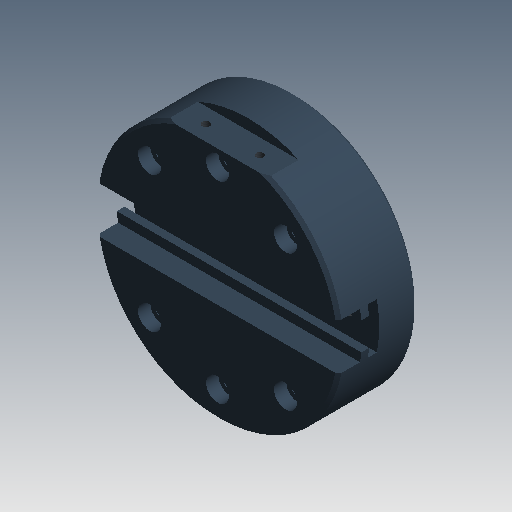
# Autodesk Inventor part: 210-101b
Saved by Autodesk Inventor 2020.1 (Build 241239000, 239)
## iProperties
Created: 2006-01-27
Part Number: 210-101b
Document SubType Name: Modeling
Designer: Kevin
Manufacturer: Standard
Standards Organization: Custom
Description: ADJUSTABLE CLAMP HEAD
Density: 1 g/cm^3
Material: Generic
Appearance: Grey - Blue Dark
Slot: 30.000 mm
Title: BLOCK
Author: Kevin
Revision Number: -
Autodesk Inventor part; units mm, degrees
ref_plane "YZ Plane" through (0, 0, 0) normal (1, 0, 0) x (0, 1, 0)
ref_plane "XZ Plane" through (0, 0, 0) normal (0, 1, 0) x (-1, 0, 0)
ref_plane "XY Plane" through (0, 0, 0) normal (0, 0, 1) x (1, 0, 0)
sketch "Sketch2" plane through (0, 0, 0) normal (0, 0, 1) x (1, 0, 0)
  circle A0 centre (0, 0) radius 80
  dimension "d0" = 160
  constraints: 1 centre point
  measures "d0" diameter of A0
extrude "Extrusion1" add sketch "Sketch2" along normal blind 50
sketch "Sketch7" plane through (0, 0, 50) normal (0, 0, 1) x (1, 0, 0)
  circle A0 centre (0, 0) radius 80 projected
  circle A1 centre (0, 0) radius 62.5 construction
  point P0 (0, 62.5)
  dimension "d48" = 125
  constraints: 2 vertical alignment, 1 coincident, 2 other
hole "Hole4" at (0, 62.5, 50) direction (0, 0, -1) diameter 9 end through all counterbore diameter 15 counterbore depth 8 clearance for "Socket Head Cap Screw" size "M8" standard "Ansi Metric M Profile"
pattern_circular "Circular Pattern2" count 8 over 360 about axis through (0, 0, 0) along (0, 0, 1) of "Hole4" skipped copies 3 7
chamfer "Chamfer1" distance 2 angle 45 1 edges at (-80, 0, 50)
sketch "Sketch9" plane through (0, 0, 0) normal (1, 0, 0) x (0, 1, 0)
  line L0 (-15, 50) -> (15, 50)
  line L1 (15, 50) -> (15, 25)
  line L2 (15, 25) -> (-15, 25)
  line L3 (-15, 25) -> (-15, 50)
  line L4 (36.6942, 50) -> (51.6942, 50) projected
  line L5 (-51.6942, 50) -> (-36.6942, 50) projected
  line L6 (-70, 50) -> (-55, 50) projected
  line L7 (-51.6942, 50) -> (-36.6942, 50) projected
  line L8 (36.6942, 50) -> (51.6942, 50) projected
  line L9 (55, 50) -> (70, 50) projected
  line L10 (0, 22.5) -> (0, 57.5) projected
  line L11 (-15, 31) -> (-9, 31)
  line L12 (-9, 31) -> (-9, 36)
  line L13 (-9, 36) -> (-15, 36)
  line L14 (-15, 36) -> (-15, 31)
  line L15 (15, 31) -> (9, 31)
  line L16 (9, 31) -> (9, 36)
  line L17 (9, 36) -> (15, 36)
  line L18 (15, 36) -> (15, 31)
  point P0 (-80, 50)
  point P1 (80, 50)
  dimension "Slot" = 30
  dimension "d76" = 15
  dimension "d77" = 25
  dimension "d78" = 6
  dimension "d79" = 5
  dimension "d81" = 6
  constraints: 24 end point, 4 parallel, 4 symmetric about line, 2 horizontal, 2 perpendicular, 1 point on line
  measures "Slot" distance between parallel lines of L1 L3
  measures "d76" distance between parallel lines of L1 L10
  measures "d77" distance of L0.end L1.end
  measures "d78" distance between parallel lines of L2 L11
  measures "d79" distance of L11.end L12.end
  measures "d81" distance between parallel lines of L12 L14
extrude "Extrusion6" cut sketch "Sketch9" along normal through all both and the other way through all contours L0 L10 L2 L3 L11 L12 L13 | L0 L1 L17 L16 L15 L2 L10
sketch "Sketch8" plane through (-78.5812, -15, 25) normal (0, 0, 1) x (1, 0, 0)
  line L0 (18.5812, 15) -> (138.5812, 15) construction
  arc A0 (0, 30) -> (0, 0) centre (78.5812, 15) ccw projected
  point P0 (38.5812, 15)
  point P1 (118.5812, 15)
  point P2 (138.5812, 15)
  dimension "d59" = 20
  dimension "d60" = 20
  dimension "d61" = 80
  dimension "d82" = 40
  constraints: 3 end point, 3 point on line, 2 coincident, 1 horizontal, 1 midpoint
  measures "d59" distance of point (38.581, 15) L0.start
  measures "d60" distance of point (138.581, 15) point (118.581, 15)
  measures "d61" distance of point (118.581, 15) point (38.581, 15)
  measures "d82" distance of A0.centre point (118.581, 15)
hole "Hole5" at (-60, 0, 25) at (-40, 0, 25) at (40, 0, 25) at (60, 0, 25) direction (0, 0, -1) diameter 6.647 end through all thread size "M8x1.25" class "6H" standard "ANSI Metric M Profile"
chamfer "Chamfer2" distance 2 angle 45 1 edges at (-80, 0, 0)
sketch "Sketch10" plane through (0, 0, 50) normal (0, 0, 1) x (1, 0, 0)
  line L0 (-76.5441, 15) -> (76.5441, 15) projected
  arc A0 (78.5812, 15) -> (-78.5812, 15) centre (0, 0) ccw projected
  line L1 (-32.7418, 72.993) -> (32.7418, 72.993)
  constraints: 2 end point, 2 point on circle, 1 parallel
extrude "Extrusion7" cut sketch "Sketch10" against normal blind 20
sketch "Sketch11" plane through (-32.7418, 72.993, 30) normal (0, 1, 0) x (1, 0, 0)
  line L0 (60.2376, -20) -> (5.2459, -20) projected
  line L1 (0, 0) -> (65.4835, 0) projected
  line L2 (32.7418, -20) -> (32.7418, 0) construction
  line L3 (50.2418, -10) -> (15.2418, -10) construction
  point P0 (32.7418, -10)
  dimension "d85" = 35
  dimension "d86" = 10
  constraints: 4 end point, 4 midpoint, 1 perpendicular
  measures "d85" distance of L3.start L3.end
  measures "d86" distance from line of L1 L3.start
hole "Hole6" at (17.5, 72.993, 40) at (-17.5, 72.993, 40) direction (0, -1, 0) diameter 4.917 depth 10 tip angle 118 thread size "M6x1" class "6H" standard "ISO Metric profile"
equation "\"d76\" = 0.5 * Slot"
equation "\"d60\" = d59"
equation "\"d82\" = 0.5 * d61"
body "Solid1"
